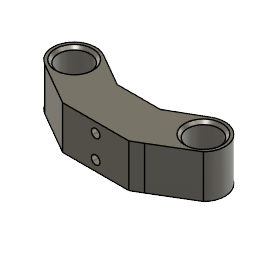
Lead scrrw double support (Autodesk Fusion 360 design; units mm, degrees)
Autodesk Fusion 360 part; units mm, degrees
sketch "Sketch1" plane through (0, 0, 0) normal (0, 1, 0) x (1, 0, 0)
  line L0 (0, 0) -> (45, 0)
  line L1 (0, 0) -> (-45, 0)
  circle A0 centre (45, 0) radius 11
  circle A1 centre (-45, 0) radius 11
  circle A2 centre (-45, 0) radius 9
  circle A3 centre (45, 0) radius 9
  line L2 (15, -30) -> (75, -30)
  line L3 (75, -30) -> (75, 30)
  line L4 (75, 30) -> (15, 30)
  line L5 (15, 30) -> (15, -30)
  line L6 (15, -30) -> (75, 30) construction
  line L7 (75, -30) -> (15, 30) construction
  line L8 (-15, 30) -> (-75, 30)
  line L9 (-75, 30) -> (-75, -30)
  line L10 (-75, -30) -> (-15, -30)
  line L11 (-15, -30) -> (-15, 30)
  line L12 (-15, 30) -> (-75, -30) construction
  line L13 (-75, 30) -> (-15, -30) construction
  line L14 (15, -30) -> (-15, -30)
  line L15 (-15, -30) -> (-15, 0)
  line L16 (-15, 0) -> (15, 0)
  line L17 (15, 0) -> (15, -30)
  circle A4 centre (-45, 0) radius 15
  circle A5 centre (45, 0) radius 15
  line L18 (-15, 0) -> (-37.5, 12.9904)
  line L19 (-15, 0) -> (-30, -25.9808)
  line L20 (-30, -25.9808) -> (-52.5, -12.9904)
  line L21 (-30, -25.9808) -> (-23.0385, -30)
  line L22 (15, 0) -> (37.5, 12.9904)
  line L23 (15, 0) -> (30, -25.9808)
  line L24 (30, -25.9808) -> (55.6066, -10.6066)
  line L25 (30, -25.9808) -> (23.0385, -30)
  line L26 (37.2058, -4.5) -> (29.7058, 8.4904)
  line L27 (-37.2058, -4.5) -> (-29.7058, 8.4904)
  line L28 (29.7058, 8.4904) -> (33.2058, 2.4282)
  line L29 (-29.7058, 8.4904) -> (-33.2058, 2.4282)
  line L30 (33.2058, 2.4282) -> (14.1532, -8.5718)
  line L31 (14.1532, -8.5718) -> (9.2043, 0)
  line L32 (-33.2058, 2.4282) -> (-14.1532, -8.5718)
  line L33 (-14.1532, -8.5718) -> (-9.2043, 0)
  point P0 (45, 0)
  point P1 (-45, 0)
  dimension "d3" = 45
  dimension "d4" = 45
  dimension "d5" = 22
  dimension "d6" = 22
  dimension "d7" = 18
  dimension "d8" = 18
  dimension "d20" = 60
  dimension "d21" = 60
  dimension "d22" = 60
  dimension "d23" = 60
  dimension "d24" = 30
  dimension "d25" = 30
  dimension "d26" = 30
  dimension "d27" = 30
  dimension "d28" = 30
  dimension "d29" = 30
  dimension "d34" = 7
  dimension "d35" = 7
  dimension "d36" = 22
  dimension "d37" = 22
  constraint coincident L0.start L1.start
  constraint horizontal L0
  constraint parallel L0 L1
  constraint coincident P0 L0.end
  constraint coincident P1 L1.end
  constraint concentric A1 A2
  constraint concentric A0 A3
  constraint horizontal L2
  constraint perpendicular L2 L3
  constraint parallel L2 L4
  constraint parallel L3 L5
  constraint coincident L6 P0
  constraint coincident L7 P0
  constraint horizontal L8
  constraint perpendicular L8 L9
  constraint parallel L8 L10
  constraint parallel L9 L11
  constraint coincident L12 P1
  constraint coincident L13 P1
  constraint horizontal L14
  constraint vertical L15
  constraint horizontal L16
  constraint vertical L17
  constraint coincident A4 L18.end
  constraint tangent A4 L18
  constraint perpendicular L18 L19
  constraint coincident A4 L20.end
  constraint tangent A4 L20
  constraint coincident L10 L21.end
  constraint perpendicular L19 L21
  constraint coincident A5 L22.end
  constraint tangent A5 L22
  constraint perpendicular L22 L23
  constraint coincident A5 L24.end
  constraint coincident L7 L24.end
  constraint coincident L2 L25.end
  constraint perpendicular L23 L25
  constraint coincident A3 L26.start
  constraint tangent A3 L26
  constraint coincident L22 L26.end
  constraint perpendicular L22 L26
  constraint coincident A2 L27.start
  constraint tangent A2 L27
  constraint coincident L18 L27.end
  constraint perpendicular L18 L27
  constraint coincident L26 L28.end
  constraint perpendicular L18 L29
  constraint perpendicular L23 L30
  constraint perpendicular L30 L31
  constraint perpendicular L19 L32
  constraint perpendicular L32 L33
  constraint coincident L0 L31.end
  constraint coincident L1 L33.end
  measures "d3" distance of L0.start P0
  measures "d4" distance of L0.start P1
  measures "d5" diameter of A0
  measures "d6" diameter of A1
  measures "d7" diameter of A2
  measures "d8" diameter of A3
  measures "d20" distance of L3.end L4.end
  measures "d21" distance of L2.end L3.end
  measures "d22" distance of L9.end L10.end
  measures "d23" distance of L8.end L9.end
  measures "d24" distance of L2.start L10.end
  measures "d25" distance of L2.start L16.end
  measures "d26" diameter of A4
  measures "d27" diameter of A5
  measures "d28" distance of L15.end L19.end
  measures "d29" distance of L16.end L23.end
  measures "d34" distance of L26.end L28.end
  measures "d35" distance of L27.end L29.end
  measures "d36" distance of L28.end L30.end
  measures "d37" distance of L29.end L32.end
extrude "Extrude3" add sketch "Sketch1" along normal blind 30 contours L0 L1 L5 L11 L14 L15 L16 L17 L30 L31 L32 L33 | L0 L5 L16 L17 L30 L31 | L1 L11 L15 L16 L32 L33 | L0 A5 L22 L26 L28 L30 | L5 L17 L23 L30 | L0 L23 L30 | L1 L19 L32 | L1 A4 L18 L27 L29 L32 | L11 L15 L19 L32 | L0 A5 L30 | L0 A5 L23 L24 L30 | L2 L5 L17 L23 L25 L30 | A5 L22 L26 L28 | L1 A4 L19 L20 L32 | L1 A4 L32 | L10 L11 L15 L19 L21 L32 | A4 L18 L27 L29 | L0 A0 A5 L26 L30 | L0 A0 A5 L24 L26 L28 | A5 L26 L28 L30 | L1 A1 A4 L27 L29 | L1 A1 A4 L27 L32 | A4 L27 L29 L32
extrude "Extrude4" add sketch "Sketch1" along normal blind 5 contours L0 A0 L26 | L0 A3 L26 | L0 A0 L26 | L1 A2 L27 | L1 A1 L27 | L1 A1 L27
extrude "Extrude5" cut sketch "Sketch1" along normal blind 21 contours L0 L5 L16 L17 L30 L31 | L1 L11 L15 L16 L32 L33 | L0 A5 L22 L26 L28 L30 | L5 L17 L23 L30 | L0 L23 L30 | L1 L19 L32 | L1 A4 L18 L27 L29 L32 | L11 L15 L19 L32 | A5 L26 L28 L30 | A4 L27 L29 L32
chamfer "Chamfer3" distance 2 angle 45 4 edges at (34.7444, 30, -3.9778) (-55.2556, 30, -3.9778) (-53.3909, 5, -3.2545) (36.6091, 5, -3.2545)
sketch "Sketch3" plane through (0, 0, 0) normal (0, 0, -1) x (-1, 0, 0)
  line L0 (-9.2043, 21) -> (-9.2043, 0)
  line L1 (-9.2043, 0) -> (9.2043, 0)
  line L2 (9.2043, 0) -> (9.2043, 21)
  line L3 (9.2043, 21) -> (15, 21)
  line L4 (15, 21) -> (15, 30)
  line L5 (15, 30) -> (-15, 30)
  line L6 (-15, 30) -> (-15, 21)
  line L7 (-15, 21) -> (-9.2043, 21)
  line L8 (0, 0) -> (0, 7)
  line L9 (0, 30) -> (0, 23)
  circle A0 centre (0, 23) radius 3
  circle A1 centre (0, 7) radius 3
  dimension "d41" = 7
  dimension "d42" = 7
  dimension "d43" = 6
  dimension "d44" = 6
  constraint coincident L8.start origin
  constraint perpendicular L5 L8
  constraint midpoint L5 L9.start
  constraint perpendicular L5 L9
  constraint coincident L9.end A0.centre
  constraint coincident L8.end A1.centre
  measures "d41" distance of L8.start L8.end
  measures "d42" distance of L9.start L9.end
  measures "d43" diameter of A0
  measures "d44" diameter of A1
extrude "Extrude6" cut sketch "Sketch3" against normal blind 30 contours A0 | A1
